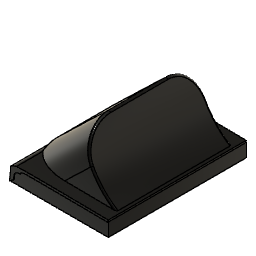
Display Part (Autodesk Fusion 360 design; units mm, degrees)
Autodesk Fusion 360 part; units mm, degrees
note: some values were not read from the file. Set by a fixed rule: which sketch regions a step uses.
sketch "Sketch1" plane through (0, 0, 0) normal (0, 1, 0) x (1, 0, 0)
  spline S0 degree 5 poles (0, 0) (0.1164, -0.2274) (0.3465, -0.7545) (0.6835, -1.7626) (1.1165, -3.5488) (1.6292, -6.5504) (2.1126, -10.3401) (2.5684, -14.8758) (2.9993, -20.0791) (3.4086, -25.8643) (3.7992, -32.1543) (4.0984, -37.544) (4.3159, -41.772) (4.4579, -44.6719) (4.5281, -46.1421) knots 0 0 0 0 0 0 0.1 0.2 0.3 0.4 0.5 0.6 0.7 0.8 0.9 1 1 1 1 1 1
  spline S1 degree 5 poles (4.5281, -46.1421) (4.8003, -46.4238) (5.3563, -46.978) (6.2248, -47.7817) (7.4531, -48.7974) (9.1133, -49.9676) (10.9083, -51.0308) (12.8467, -51.9797) (14.9298, -52.8137) (17.1481, -53.54) (19.4898, -54.1682) (21.4529, -54.5993) (22.9725, -54.8851) (24.0062, -55.0592) (24.5281, -55.1421) knots 0 0 0 0 0 0 0.1 0.2 0.3 0.4 0.5 0.6 0.7 0.8 0.9 1 1 1 1 1 1
  spline S2 degree 5 poles (24.5281, -55.1421) (25.0432, -55.3124) (26.7537, -55.631) (31.3608, -56.0434) (41.65, -56.4601) (61.5654, -56.7544) (88.1118, -56.8357) (120.5177, -56.7289) (157.928, -56.4612) (199.5405, -56.0586) (244.7035, -55.542) (283.3076, -55.0492) (313.5378, -54.6386) (334.2496, -54.347) (344.7451, -54.1967) knots 0 0 0 0 0 0 0.1 0.2 0.3 0.4 0.5 0.6 0.7 0.8 0.9 1 1 1 1 1 1
  line L0 (344.7451, -54.1967) -> (342.8805, -46.3082)
  spline S3 degree 5 poles (342.8805, -46.3082) (333.1773, -46.4031) (314.0218, -46.5882) (286.0411, -46.8518) (250.2636, -47.1746) (208.3293, -47.526) (169.6204, -47.8171) (134.7778, -48.0359) (104.6118, -48.1673) (80.0398, -48.1941) (61.9418, -48.0999) (53.1976, -47.9173) (49.9094, -47.7192) (49.1421, -47.5605) (49.1149, -47.4745) knots 0 0 0 0 0 0 0.1 0.2 0.3 0.4 0.5 0.6 0.7 0.8 0.9 1 1 1 1 1 1
  spline S4 degree 5 poles (49.1149, -47.4745) (48.742, -47.3855) (48.0095, -47.2018) (46.9507, -46.9095) (45.6205, -46.4856) (44.1031, -45.8943) (42.7465, -45.2353) (41.5677, -44.5013) (40.5821, -43.6861) (39.7931, -42.7879) (39.1911, -41.8111) (38.849, -40.9708) (38.6664, -40.3094) (38.577, -39.8548) (38.5404, -39.6242) knots 0 0 0 0 0 0 0.1 0.2 0.3 0.4 0.5 0.6 0.7 0.8 0.9 1 1 1 1 1 1
  spline S5 degree 5 poles (38.5404, -39.6242) (38.0967, -39.6221) (37.2141, -39.6065) (35.9045, -39.549) (34.1877, -39.4031) (32.0938, -39.0975) (30.0568, -38.6573) (28.0813, -38.0714) (26.1703, -37.3331) (24.3214, -36.4477) (22.53, -35.4261) (21.1393, -34.5087) (20.1185, -33.7678) (19.4477, -33.2509) (19.1148, -32.9866) knots 0 0 0 0 0 0 0.1 0.2 0.3 0.4 0.5 0.6 0.7 0.8 0.9 1 1 1 1 1 1
  spline S6 degree 5 poles (19.1148, -32.9866) (19.0167, -32.9268) (18.8222, -32.7654) (18.5354, -32.3981) (18.163, -31.6538) (17.715, -30.2806) (17.2849, -28.4541) (16.8717, -26.1991) (16.4736, -23.5611) (16.0887, -20.5894) (15.7152, -17.3284) (15.4245, -14.5148) (15.2106, -12.2981) (15.0699, -10.7738) (15, -10) knots 0 0 0 0 0 0 0.1 0.2 0.3 0.4 0.5 0.6 0.7 0.8 0.9 1 1 1 1 1 1
  spline S7 degree 5 poles (15, -10) (14.7697, -9.8933) (14.3027, -9.6711) (13.5827, -9.312) (12.5834, -8.7805) (11.2646, -8.0229) (9.8712, -7.1655) (8.3993, -6.2031) (6.8507, -5.1381) (5.2314, -3.9785) (3.5484, -2.7336) (2.1558, -1.676) (1.0872, -0.8504) (0.3641, -0.2858) (0, 0) knots 0 0 0 0 0 0 0.1 0.2 0.3 0.4 0.5 0.6 0.7 0.8 0.9 1 1 1 1 1 1
  line L1 (0, 0) -> (342.8805, 0)
  line L2 (342.8805, 0) -> (342.8805, -46.3082)
  spline S8 degree 5 poles (21.864, -54.665) (21.8945, -54.7724) (21.9571, -55.01) (22.0561, -55.4349) (22.1985, -56.1407) (22.3946, -57.2668) (22.6096, -58.648) (22.8434, -60.2815) (23.0943, -62.146) (23.3604, -64.2159) (23.64, -66.4663) (23.8732, -68.3953) (24.0531, -69.9093) (24.1752, -70.9479) (24.2367, -71.4745) knots 0 0 0 0 0 0 0.1 0.2 0.3 0.4 0.5 0.6 0.7 0.8 0.9 1 1 1 1 1 1
  spline S9 degree 5 poles (210, -250) (211.2902, -244.5713) (213.9705, -233.8422) (218.2908, -218.1331) (224.661, -197.9699) (233.7118, -174.1618) (243.958, -151.8871) (255.5143, -131.2932) (268.4707, -112.4954) (282.8164, -95.4799) (298.4649, -80.1357) (311.9497, -69.0995) (322.5736, -61.477) (329.8792, -56.6815) (333.5878, -54.3553) knots 0 0 0 0 0 0 0.1 0.2 0.3 0.4 0.5 0.6 0.7 0.8 0.9 1 1 1 1 1 1
  line L3 (210, -250) -> (24.2367, -71.4745)
  point P0 (1.7078, -7.3473)
  point P1 (12.1883, -51.6322)
  point P2 (46.0718, -56.4651)
  point P3 (59, -48)
  point P4 (41, -44)
  point P5 (28, -38)
  point P6 (17.6514, -29.9134)
  point P7 (9.3099, -6.7914)
  point P8 (22.5281, -58.1421)
  point P9 (260.158, -125.0797)
  constraint coincident S0.start S7.end
  constraint horizontal L1
  constraint perpendicular L1 L2
  constraint coincident S1 S8.start
  constraint coincident S2 S9.end
extrude "Extrude1" add sketch "Sketch1" along normal blind 480 contours S0 S1 S2 L0 S3 S4 S5 S6 S7 makes body 1
extrude "Extrude2" add sketch "Sketch1" along normal blind 482 and the other way blind -2 contours S3 S4 S5 S6 S7 L1 L2 bodies 1
extrude "Extrude3" add sketch "Sketch1" along normal blind 400 separate body contours S1 S2 S8 S9 L3 makes body 2
move_body "Move1" bodies 2 to x (1, 0, 0) y (0, 1, 0) z (0, 0, 1) at (0, 40, 0)
fillet "Fillet1" radius 100 1 edges at (117.1184, 440, 160.7373) on bodies 2
fillet "Fillet2" radius 100 1 edges at (117.1184, 40, 160.7373) on bodies 2
sketch "Sketch1 (2)" plane through (0, 0, 0) normal (0, 1, 0) x (1, 0, 0) in component "Display"
  line L0 (-203.3576, -180.502) -> (-129.014, -180.502)
  line L1 (-129.014, -180.502) -> (-129.014, -80.1792)
  line L2 (-129.014, -80.1792) -> (-203.3576, -80.1792)
  line L3 (-203.3576, -80.1792) -> (-203.3576, -180.502)
  dimension "d13" = 74.3436
  dimension "d14" = 100.3228
  constraint horizontal L0
  constraint vertical L1
  constraint horizontal L2
  constraint vertical L3
  measures "d13" distance of L0.start L0.end
  measures "d14" distance of L0.start L2.end
copy_body "CutPasteBodies1" bodies 1 2 removing the originals makes body 3 makes body 4 in component "Display"
fillet "Fillet1'" radius 5 5 edges at (285.0467, 440, 93.8649) (218.9614, 411.623, 216.7083) (210, 240, 250) (218.9559, 68.3942, 216.7273) (285.0467, 40, 93.8649) on bodies 4 in component "Display"
scale "Scale1" factor 0.75 about (0, 0, 0) bodies 3 4 in component "Display"
component "Display" placed x (1, 0, 0) y (0, 1, 0) z (0, 0, 1) at (0, 0, 0)
